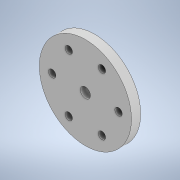
# Autodesk Inventor part: flange2
Saved by Autodesk Inventor 2022 (Build 260153000, 153)
## iProperties
Created: 2022-03-15
Part Number: flange2
Material: Generic
Document SubType Name: Modeling
Designer: karee
Density: 1 g/cm^3
Appearance: Default
Author: karee
Autodesk Inventor part; units mm, degrees
ref_plane "YZ Plane" through (0, 0, 0) normal (1, 0, 0) x (0, 1, 0)
ref_plane "XZ Plane" through (0, 0, 0) normal (0, 1, 0) x (-1, 0, 0)
sketch "Sketch1" plane through (0, 0, 0) normal (0, 0, 1) x (1, 0, 0)
  circle A0 centre (0, 0) radius 50
  dimension "d1" = 100
  constraints: 1 centre point, 1 coincident
  measures "d1" diameter of A0
extrude "Extrusion1" add sketch "Sketch1" along normal blind 370
ref_plane "Work Plane1" through (0, 0, 360) normal (0, 0, 1) x (1, 0, 0)
sketch "Sketch2" plane through (0, 0, 360) normal (0, 0, 1) x (1, 0, 0)
  point P0 (0, 0)
sketch "Sketch3" plane through (0, 0, 360) normal (0, 0, 1) x (1, 0, 0)
  circle A0 centre (0, 0) radius 50
  constraints: 1 centre point, 1 coincident
extrude "Extrusion2" cut sketch "Sketch3" against normal blind 370
sketch "Sketch4" plane through (0, 0, 370) normal (0, 0, 1) x (1, 0, 0)
  circle A0 centre (0, 0) radius 5.5
  line L0 (0, 0) -> (36, 0)
  circle A1 centre (36, 0) radius 4
  dimension "d7" = 11
  dimension "d8" = 36
  dimension "d9" = 8
  constraints: 2 centre point, 2 coincident, 2 end point, 1 horizontal
  measures "d7" diameter of A0
  measures "d8" distance of L0.start L0.end
  measures "d9" diameter of A1
extrude "Extrusion3" cut sketch "Sketch4" against normal blind 370 contours A0
sketch "Sketch5" plane through (0, 0, 370) normal (0, 0, 1) x (1, 0, 0)
  line L0 (0, 0) -> (36, 0)
  circle A0 centre (36, 0) radius 4
  dimension "d12" = 36
  dimension "d13" = 8
  constraints: 2 end point, 1 centre point, 1 coincident, 1 horizontal
  measures "d12" distance of L0.start L0.end
  measures "d13" diameter of A0
extrude "Extrusion4" cut sketch "Sketch5" against normal blind 370
pattern_circular "Circular Pattern1" count 6 over 360 about axis through (0, 0, 370) along (0, 0, -1) of "Extrusion4"
body "Solid1"
